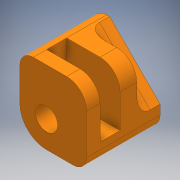
# Autodesk Inventor part: Plate Adapter 2.0
Saved by Autodesk Inventor 2017 (Build 210142000, 142)
## iProperties
Created: 2017-04-02
Part Number: Plate Adapter 2.0
Material: Generic
Document SubType Name: Modeling
Designer: gilef
Density: 1 g/cm^3
Appearance: Orange
Author: gilef
Autodesk Inventor part; units mm, degrees
ref_plane "YZ Plane" through (0, 0, 0) normal (1, 0, 0) x (0, 1, 0)
ref_plane "XZ Plane" through (0, 0, 0) normal (0, 1, 0) x (-1, 0, 0)
ref_plane "XY Plane" through (0, 0, 0) normal (0, 0, 1) x (1, 0, 0)
sketch "Sketch1" plane through (0, 0, 0) normal (0, 1, 0) x (-1, 0, 0)
  line L0 (0, 0) -> (0, -5)
  arc A0 (-3, -8) -> (0, -5) centre (-3, -5) ccw
  line L1 (-3, -8) -> (-8, -8)
  line L2 (-8, -8) -> (0, 0)
  line L3 (0, 0) -> (2, 0)
  line L4 (2, 0) -> (2, -7)
  arc A1 (-2, -11) -> (2, -7) centre (-2, -7) ccw
  line L5 (-8, -11) -> (-2, -11)
  line L6 (-8, -11) -> (-8, -8)
  dimension "d0" = 5
  dimension "d1" = 3
  dimension "d2" = 4
  dimension "d3" = 3
  dimension "d11" = 2
  constraints: 14 end point, 4 point on circle, 4 tangent, 3 horizontal, 3 vertical, 2 centre point, 1 perpendicular
  measures "d0" distance of L0.start L0.end
  measures "d1" radius of A0
  measures "d2" radius of A1
  measures "d3" distance of L5.start L1.end
  measures "d11" distance of L0.start L3.end
extrude "Extrusion1" add sketch "Sketch1" along normal blind 5.5 contours L3 L4 A1 L5 L6 L1 A0 L0
sketch "Sketch2" plane through (0, 5.5, 0) normal (0, 1, 0) x (1, 0, 0)
  line L0 (0, 0) -> (0, 5) projected
  arc A0 (3, 8) -> (0, 5) centre (3, 5) ccw projected
  line L1 (3, 8) -> (8, 8) projected
  line L2 (0, 0) -> (8, 8)
  line L3 (0, 0) -> (0, 5)
  line L4 (8, 8) -> (3, 8)
  arc A1 (3, 8) -> (0, 5) centre (3, 5) ccw
  line L5 (8, 8) -> (8, 3)
  line L6 (0, 0) -> (5, 0)
  arc A2 (5, 0) -> (8, 3) centre (5, 3) ccw
  constraints: 10 end point, 6 point on circle, 2 centre point, 2 horizontal, 2 perpendicular, 2 tangent, 2 vertical
extrude "Extrusion2" add sketch "Sketch2" against normal blind 0.5 and the other way blind 2
sketch "Sketch3" plane through (0, 0, 0) normal (0, -1, 0) x (1, 0, 0)
  line L0 (0, 0) -> (0, -5) projected
  arc A0 (0, -5) -> (3, -8) centre (3, -5) ccw projected
  line L1 (3, -8) -> (8, -8) projected
  line L2 (8, -8) -> (0, 0) projected
  line L3 (0, 0) -> (8, -8)
  line L4 (8, -8) -> (3, -8)
  line L5 (0, 0) -> (0, -5)
  arc A1 (0, -5) -> (3, -8) centre (3, -5) ccw projected
  arc A2 (0, -5) -> (0, -5) centre (6.2395, -3.6998) ccw
  arc A3 (0, -5) -> (3, -8) centre (3, -5) ccw
  line L6 (8, -8) -> (8, -3)
  arc A4 (8, -3) -> (5, 0) centre (5, -3) ccw
  line L7 (0, 0) -> (5, 0)
  constraints: 10 end point, 4 point on circle, 3 tangent, 2 centre point, 2 collinear, 2 vertical, 1 horizontal, 1 perpendicular, 4 other
extrude "Extrusion3" add sketch "Sketch3" against normal blind 2 contours L2 A2 L0 | L7 A2 L2 | A2 L2 L1 A0 L0 | A2 L7 A4 L6 L2 | A2 A0
fillet "Fillet1" radius 2 2 edges at (-2, 2.75, 0) (8, 2.75, -11)
sketch "Sketch5" plane through (0, 5.5, 0) normal (0, 1, 0) x (1, 0, 0)
  circle A0 centre (2, 7) radius 1.6667
  line L0 (6, 11) -> (2, 11) projected
  line L1 (-2, 7) -> (-2, 2) projected
  point P0 (0, 0)
  dimension "d12" = 3.3333
  constraints: 1 centre point, 1 other
  measures "d12" diameter of A0
sketch "Sketch7" plane through (0, 5.5, 0) normal (0, 1, 0) x (1, 0, 0)
  arc A0 (2, 11) -> (-2, 7) centre (2, 7) ccw projected
  line L0 (-0.3678, 9.3678) -> (2.8667, 10.2345)
  line L1 (2.8667, 10.2345) -> (5.2345, 7.8667)
  line L2 (5.2345, 7.8667) -> (4.3678, 4.6322)
  line L3 (4.3678, 4.6322) -> (1.1333, 3.7655)
  line L4 (1.1333, 3.7655) -> (-1.2345, 6.1333)
  line L5 (-1.2345, 6.1333) -> (-0.3678, 9.3678)
  arc A1 (2, 11) -> (-2, 7) centre (2, 7) ccw projected
  line L6 (0, 0) -> (8, 8) projected
  line L7 (-1.2345, 6.1333) -> (-1.9987, 6.8975)
  line L8 (2.8667, 10.2345) -> (2.1025, 10.9987)
  line L9 (6, 11) -> (2, 11) projected
  arc A2 (-2, 2) -> (0, 0) centre (0, 2) ccw projected
  line L10 (8, 8) -> (8, 9) projected
  arc A3 (8, 9) -> (6, 11) centre (6, 9) ccw projected
  line L11 (8, 8) -> (0, 0) projected
  arc A4 (-2, 2) -> (0, 0) centre (0, 2) ccw
  line L12 (-2, 7) -> (-2, 2) projected
  line L13 (0, 0) -> (8, 8)
  line L14 (8, 9) -> (8, 8)
  arc A5 (8, 9) -> (6, 11) centre (6, 9) ccw projected
  arc A6 (8, 9) -> (6, 11) centre (6, 9) ccw
  line L15 (2.1025, 10.9987) -> (6, 11)
  line L16 (-2, 7) -> (-2, 2) projected
  line L17 (-1.9987, 6.8975) -> (-2, 2)
  dimension "d15" = 5.8
  constraints: 24 end point, 8 point on circle, 3 collinear, 2 centre point, 2 coincident, 2 tangent, 1 parallel, 1 perpendicular, 13 other
  measures "d15" distance between parallel lines of L1 L4
extrude "Extrusion8" add sketch "Sketch7" along normal blind 5.5 contours L9 A3 L10 L6 A2 L12 L7 L4 L3 L2 L1 L8
sketch "Sketch11" plane through (0, 11, 0) normal (0, 1, 0) x (1, 0, 0)
  line L0 (2.1025, 10.9987) -> (5.2345, 7.8667) projected
  line L1 (5.2345, 7.8667) -> (4.3678, 4.6322) projected
  line L2 (4.3678, 4.6322) -> (1.1333, 3.7655) projected
  line L3 (1.1333, 3.7655) -> (-1.9987, 6.8975) projected
  line L4 (4.3678, 4.6322) -> (1.1333, 3.7655)
  line L5 (1.1333, 3.7655) -> (-1.2345, 6.1333)
  line L6 (-1.2345, 6.1333) -> (-0.3678, 9.3678)
  line L7 (-0.3678, 9.3678) -> (2.8667, 10.2345)
  line L8 (2.8667, 10.2345) -> (5.2345, 7.8667)
  line L9 (5.2345, 7.8667) -> (4.3678, 4.6322)
  arc A0 (2, 11) -> (-2, 7) centre (2, 7) ccw projected
  line L10 (2.8667, 10.2345) -> (2.1025, 10.9987)
  line L11 (6, 11) -> (2, 11) projected
  line L12 (2.1025, 10.9987) -> (2, 11)
  line L13 (-1.2345, 6.1333) -> (-1.9987, 6.8975)
  line L14 (-2, 7) -> (-2, 2) projected
  line L15 (-2, 7) -> (-1.9987, 6.8975)
  arc A1 (2, 11) -> (-2, 7) centre (2, 7) ccw projected
  arc A2 (2, 11) -> (-2, 7) centre (2, 7) ccw
  point P0 (0, 0)
  point P1 (2, 7)
  constraints: 20 end point, 2 collinear, 2 point on circle, 1 centre point, 1 concentric, 13 other
extrude "Extrusion10" add sketch "Sketch11" against normal through all contours L0 L7 L6 L3 L14 A0 L11
sketch "Sketch12" plane through (0, 11, 0) normal (0, 1, 0) x (1, 0, 0)
  line L0 (1.1333, 3.7655) -> (-1.2345, 6.1333) projected
  line L1 (4.3678, 4.6322) -> (1.1333, 3.7655) projected
  line L2 (5.2345, 7.8667) -> (4.3678, 4.6322) projected
  line L3 (2.8667, 10.2345) -> (5.2345, 7.8667) projected
  line L4 (-0.3678, 9.3678) -> (2.8667, 10.2345) projected
  line L5 (-1.2345, 6.1333) -> (-0.3678, 9.3678) projected
  point P0 (0, 0)
extrude "Extrusion11" add sketch "Sketch12" against normal blind 6
extrude "Extrusion12" cut sketch "Sketch5" along normal through all both and the other way through all
fillet "Fillet3" radius 0.25 1 edges at (0.3333, 11, -7)
sketch "Sketch14" plane through (8, 7.5, -8) normal (0.7071068, 0, 0.7071068) x (0.7071068, 0, -0.7071068)
  line L0 (0, 0) -> (0, 3.5) projected
  line L1 (-11.3137, -2) -> (-11.3137, 3.5) projected
  line L2 (0, 0) -> (-11.3137, 0)
  line L3 (-11.3137, 0) -> (-11.3137, 3.5)
  line L4 (-11.3137, 3.5) -> (0, 3.5)
  line L5 (0, 3.5) -> (0, 0)
  point P0 (-11.3137, -7.5)
  constraints: 8 end point, 2 parallel, 1 horizontal, 1 perpendicular
extrude "Extrusion14" add sketch "Sketch14" along normal blind 0.3
sketch "Sketch15" plane through (0, 7.5, 0) normal (0, -1, 0) x (1, 0, 0)
  line L0 (0, 0) -> (0.4243, 0)
  line L1 (8.2121, -7.7879) -> (0.2121, 0.2121) projected
  line L2 (0.2121, 0.2121) -> (0, 0)
  constraints: 4 end point, 1 horizontal, 1 perpendicular, 1 point on line
extrude "Extrusion15" cut sketch "Sketch15" against normal through all
sketch "Sketch16" plane through (8, 7.5, -8) normal (0, -1, 0) x (1, 0, 0)
  line L0 (0.2121, 0.2121) -> (-7.5757, 8) projected
  line L1 (0, 0) -> (0.2121, 0.2121)
  line L2 (0.2121, 0.2121) -> (0, 0.4243)
  line L3 (0, 0) -> (0, 0.4243)
  point P0 (-8, 8)
  constraints: 6 end point, 1 perpendicular, 1 point on line, 1 vertical
extrude "Extrusion16" cut sketch "Sketch16" against normal through all
fillet "Fillet5" radius 2 1 edges at (4.2121, 7.5, -3.7879)
body "Solid1"
